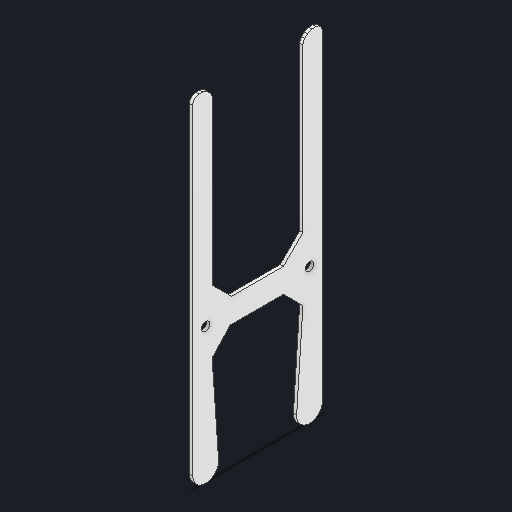
# Autodesk Inventor part: Ring Guard
Saved by Autodesk Inventor 2025.1 (Build 291241000, 241)
## iProperties
Created: 2024-11-12
Part Number: Ring Guard
Material: Acetal Resin, White
Document SubType Name: Modeling
Designer: avere
Density: 1.425 g/cm^3
Appearance: Smooth - White
Author: avere
Autodesk Inventor part; units mm, degrees
ref_plane "YZ Plane" through (0, 0, 0) normal (1, 0, 0) x (0, 1, 0)
ref_plane "XZ Plane" through (0, 0, 0) normal (0, 1, 0) x (-1, 0, 0)
ref_plane "XY Plane" through (0, 0, 0) normal (0, 0, 1) x (1, 0, 0)
sketch "Sketch1" plane through (0, 0, 0) normal (1, 0, 0) x (0, 1, 0)
  circle A0 centre (0, 0) radius 2.0955
  line L0 (0, 6.35) -> (76.2, 6.35)
  circle A1 centre (0, -50.8) radius 2.0955
  line L1 (-59.2019, -57.15) -> (76.2, -57.15)
  line L2 (76.2, 6.35) -> (96.8375, 6.35)
  line L3 (100.0125, 3.175) -> (100.0125, 1.3151)
  line L4 (95.5224, -3.175) -> (76.1708, -3.175)
  line L5 (76.1708, -47.625) -> (95.5224, -47.625)
  line L6 (100.0125, -52.1151) -> (100.0125, -53.975)
  line L7 (96.8375, -57.15) -> (76.2, -57.15)
  line L8 (99.0826, -0.9299) -> (97.7674, -2.2451)
  line L9 (97.7674, -48.5549) -> (99.0826, -49.8701)
  arc A2 (100.0125, 3.175) -> (96.8375, 6.35) centre (96.8375, 3.175) ccw
  arc A3 (99.0826, -0.9299) -> (100.0125, 1.3151) centre (96.8375, 1.3151) ccw
  arc A4 (95.5224, -3.175) -> (97.7674, -2.2451) centre (95.5224, 0) ccw
  arc A5 (97.7674, -48.5549) -> (95.5224, -47.625) centre (95.5224, -50.8) ccw
  arc A6 (100.0125, -52.1151) -> (99.0826, -49.8701) centre (96.8375, -52.1151) ccw
  arc A7 (96.8375, -57.15) -> (100.0125, -53.975) centre (96.8375, -53.975) ccw
  line L10 (59.0099, -3.175) -> (76.1708, -3.175)
  line L11 (76.1708, -47.625) -> (59.0099, -47.625)
  line L12 (0, 6.35) -> (-60.325, 6.35)
  arc A8 (-60.325, 6.35) -> (-59.8788, -6.3343) centre (-60.325, 0) ccw
  arc A9 (-59.8927, -44.5648) -> (-59.2019, -57.15) centre (-60.325, -50.9001) ccw
  line L13 (6.35, -12.7) -> (6.35, -38.1)
  line L14 (-5.5228, -38.1) -> (-5.5228, -12.0308)
  line L15 (-59.8788, -6.3343) -> (-15.0243, -3.175)
  line L16 (15.875, -3.175) -> (59.0099, -3.175)
  line L17 (-54.8848, -47.625) -> (-15.0478, -47.625)
  line L18 (15.875, -47.625) -> (59.0099, -47.625)
  line L19 (15.875, -3.175) -> (6.35, -12.7)
  line L20 (6.35, -38.1) -> (15.875, -47.625)
  line L21 (-5.5228, -38.1) -> (-15.0478, -47.625)
  line L22 (-15.0243, -3.175) -> (-5.5228, -12.0308)
  line L23 (-15.0478, -47.625) -> (-59.8927, -44.5648)
  point P0 (5.4993, -3.175)
  point P1 (0, -57.15)
  point P2 (5.4993, -47.625)
  point P3 (100.0125, -3.175)
  point P4 (100.0125, -47.625)
  point P5 (100.0125, -57.15)
  point P6 (100.0125, 0)
  point P7 (96.8375, -3.175)
  point P8 (96.8375, -47.625)
  point P9 (100.0125, -50.8)
  point P10 (38.1, 6.35)
  point P11 (-5.5228, -2.5058)
  point P12 (-5.5228, -47.625)
  point P13 (85.8466, -3.175)
  point P14 (6.35, -3.175)
  point P15 (6.35, -47.625)
  dimension "d0" = 4.191
  dimension "d6" = 4.191
  dimension "d15" = 3.175
  dimension "d16" = 3.175
  dimension "d17" = 3.175
  dimension "d18" = 3.175
  dimension "d19" = 3.175
  dimension "d29" = 9.525
  dimension "d30" = 9.525
  dimension "d31" = 9.525
  dimension "d32" = 9.525
  dimension "d33" = 9.525
  dimension "d34" = 9.525
  dimension "d35" = 9.525
  dimension "d36" = 9.525
  dimension "d37" = 9.525
  dimension "d38" = 9.525
  dimension "d39" = 12.7
  dimension "d40" = 12.7
  constraints: 48 end point, 25 point on line, 16 point on circle, 14 tangent, 10 centre point, 8 horizontal, 5 equal radius, 5 perpendicular, 3 parallel, 2 midpoint, 1 coincident, 1 vertical, 3 other
  measures "d0" diameter of A0
  measures "d6" diameter of A1
  measures "d15" distance of point (100.013, 0) point (100.013, -3.175)
  measures "d16" distance of point (96.838, -3.175) point (100.013, -3.175)
  measures "d17" distance of point (96.838, -47.625) point (100.013, -47.625)
  measures "d18" distance of point (100.012, -50.8) point (100.013, -47.625)
  measures "d19" radius of A2
  measures "d29" distance from line of L2 point (85.847, -3.175)
  measures "d30" distance between parallel lines of L7 L5
  measures "d31" distance of L16.start point (6.35, -3.175)
  measures "d32" distance of L13.start point (6.35, -3.175)
  measures "d33" distance of L13.end point (6.35, -47.625)
  measures "d34" distance of L18.start point (6.35, -47.625)
  measures "d35" distance of L14.start point (-5.523, -47.625)
  measures "d36" distance of L17.end point (-5.523, -47.625)
  measures "d37" distance of L15.end point (-5.523, -2.506)
  measures "d38" distance of L14.end point (-5.523, -2.506)
  measures "d39" diameter of A8
  measures "d40" diameter of A9
extrude "Extrusion1" add sketch "Sketch1" along normal blind 1.5875
feature "Bend Part1" [suppressed]
feature "Bend Part2" [suppressed]
equation "\"d15\" = d7"
equation "\"d16\" = d15"
equation "\"d17\" = d7"
equation "\"d18\" = d17"
equation "\"d32\" = d31"
equation "\"d33\" = d31"
equation "\"d34\" = d33"
equation "\"d35\" = d31"
equation "\"d36\" = d35"
equation "\"d37\" = d31"
equation "\"d38\" = d37"
equation "\"d7\" = 3.175"
body "Solid1"
